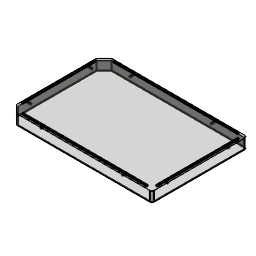
GREINER 96 WELL PLATE LID (Created) (Autodesk Fusion 360 design; units mm, degrees)
part number: 2026-02-05-10-27-23-618
Autodesk Fusion 360 part; units mm, degrees
sketch "Sketch1" plane through (0, 0, 0) normal (0, 0, 1) x (1, 0, 0)
  line L0 (61.42, -42.3) -> (-56.55, -42.3)
  line L1 (-63.55, -35.3) -> (-63.55, 35.3)
  line L2 (-56.55, 42.3) -> (61.42, 42.3)
  line L3 (63.55, 40.17) -> (63.55, -40.17)
  line L4 (63.55, -42.3) -> (-63.55, 42.3) construction
  line L5 (-63.55, -42.3) -> (63.55, 42.3) construction
  line L6 (-56.55, 42.3) -> (-63.55, 35.3)
  line L7 (0, -42.3) -> (0, 42.3) construction
  line L8 (63.55, 0) -> (-63.55, 0) construction
  line L9 (-56.55, -42.3) -> (-63.55, -35.3)
  arc A0 (63.55, 40.17) -> (61.42, 42.3) centre (61.42, 40.17) ccw
  arc A1 (61.42, -42.3) -> (63.55, -40.17) centre (61.42, -40.17) ccw
  dimension "d1" = 84.6
  dimension "d2" = 127.1
  dimension "d3" = 7
  dimension "d4" = 7
  dimension "d5" = 2.13
  constraint horizontal L0
  constraint perpendicular L0 L1
  constraint parallel L0 L2
  constraint parallel L1 L3
  constraint coincident L4 origin
  constraint coincident L5 origin
  constraint coincident L4.end L2
  constraint coincident L4.end L1
  constraint coincident L2 L7.end
  constraint perpendicular L2 L7
  constraint coincident L1 L8.end
  constraint perpendicular L1 L8
  constraint symmetric L2.start L8 L0.end
  constraint symmetric L1.end L8 L1.start
  constraint coincident L0 L7.start
  constraint coincident L3 L8.start
  constraint coincident L5.end L2
  constraint coincident L5.end L3
  constraint tangent L2 A0
  constraint tangent L3 A0
  constraint symmetric L8 L2.end L0.start
  constraint symmetric L8 L3.start L3.end
  constraint symmetric L8 A0 A1
  measures "d1" distance of L5.start L4.end
  measures "d2" distance of L4.end L5.end
  measures "d3" distance of L4.end L2.start
  measures "d4" distance of L4.end L1.end
  measures "d5" radius of A0
extrude "Extrude1" add sketch "Sketch1" against normal blind 9
sketch "Sketch2" plane through (0, 0, -9) normal (0, 0, -1) x (1, 0, 0)
  line L0 (61.42, 42.3) -> (-56.55, 42.3)
  line L1 (-56.55, 42.3) -> (-63.55, 35.3)
  line L2 (-63.55, 35.3) -> (-63.55, -35.3)
  line L3 (-63.55, -35.3) -> (-56.55, -42.3)
  line L4 (-56.55, -42.3) -> (61.42, -42.3)
  arc A0 (61.42, -42.3) -> (63.55, -40.17) centre (61.42, -40.17) ccw
  line L5 (63.55, -40.17) -> (63.55, 40.17)
  arc A1 (63.55, 40.17) -> (61.42, 42.3) centre (61.42, 40.17) ccw
  line L6 (61.42, -41.3) -> (-56.1358, -41.3)
  line L7 (-62.55, -34.8858) -> (-62.55, 34.8858)
  line L8 (-56.1358, 41.3) -> (61.42, 41.3)
  line L9 (62.55, 40.17) -> (62.55, -40.17)
  line L10 (62.55, -41.3) -> (-62.55, 41.3) construction
  line L11 (-62.55, -41.3) -> (62.55, 41.3) construction
  line L12 (-56.1358, 41.3) -> (-62.55, 34.8858)
  arc A2 (62.55, 40.17) -> (61.42, 41.3) centre (61.42, 40.17) ccw
  line L13 (63.55, 0) -> (-63.55, 0) construction
  line L14 (-56.1358, -41.3) -> (-62.55, -34.8858)
  arc A3 (61.42, -41.3) -> (62.55, -40.17) centre (61.42, -40.17) ccw
  dimension "d8" = 125.1
  dimension "d9" = 82.6
  dimension "d10" = 6.4142
  dimension "d11" = 6.4142
  dimension "d12" = 1
  dimension "d13" = 1.13
  constraint horizontal L6
  constraint perpendicular L6 L7
  constraint parallel L6 L8
  constraint parallel L7 L9
  constraint coincident L10 origin
  constraint coincident L11 origin
  constraint coincident L10.end L8
  constraint coincident L10.end L7
  constraint coincident L11.end L9
  constraint coincident L11.end L8
  constraint tangent L9 A2
  constraint tangent L8 A2
  constraint midpoint L5 L13.start
  constraint midpoint L2 L13.end
  constraint symmetric L8.start L13 L6.end
  constraint symmetric L7.end L13 L7.start
  constraint symmetric L9.start L13 L9.end
  constraint symmetric L8.end L13 L6.start
  constraint symmetric A2 L13 A3
  measures "d8" distance of L10.end L11.end
  measures "d9" distance of L11.start L10.end
  measures "d10" distance of L10.end L8.start
  measures "d11" distance of L10.end L7.end
  measures "d12" distance of L1 L12
  measures "d13" radius of A2
extrude "Extrude2" cut sketch "Sketch2" against normal blind 8 contours L6 L7 L8 L9 L12 A2 L14 A3
sketch "Sketch3" plane through (0, 0, -1) normal (0, 0, -1) x (1, 0, 0)
  line L0 (-56.1358, -41.3) -> (61.42, -41.3)
  arc A0 (61.42, -41.3) -> (62.55, -40.17) centre (61.42, -40.17) ccw
  line L1 (62.55, -40.17) -> (62.55, 40.17)
  arc A1 (62.55, 40.17) -> (61.42, 41.3) centre (61.42, 40.17) ccw
  line L2 (61.42, 41.3) -> (-56.1358, 41.3)
  line L3 (-56.1358, 41.3) -> (-62.55, 34.8858)
  line L4 (-62.55, 34.8858) -> (-62.55, -34.8858)
  line L5 (-62.55, -34.8858) -> (-56.1358, -41.3)
  line L6 (-62.55, 32.8642) -> (-35.55, 32.8642) construction
  line L7 (-35.55, 32.8642) -> (-35.55, 41.3) construction
  line L8 (-35.55, 41.3) -> (-36.55, 41.3)
  line L9 (-36.55, 41.3) -> (-36.55, 37.5)
  line L10 (-36.55, 37.5) -> (-35.55, 37.5)
  line L11 (-35.55, 37.5) -> (-35.55, 41.3)
  line L12 (-50.2731, 41.3) -> (-50.2731, 26.6) construction
  line L13 (-50.2731, 26.6) -> (-62.55, 26.6) construction
  line L14 (-62.55, 26.6) -> (-58.75, 26.6)
  line L15 (-58.75, 26.6) -> (-58.75, 27.6)
  line L16 (-58.75, 27.6) -> (-62.55, 27.6)
  line L17 (-62.55, 27.6) -> (-62.55, 26.6)
  line L18 (62.55, 0) -> (-62.55, 0) construction
  line L19 (-62.55, 30.673) -> (-62.55, 55) construction
  line L20 (62.55, 34.8173) -> (62.55, 55) construction
  line L21 (62.55, 55) -> (-62.55, 55) construction
  line L22 (0, 55) -> (0, -41.3) construction
  line L23 (62.55, 27.6) -> (62.55, 26.6)
  line L24 (62.55, 26.6) -> (58.75, 26.6)
  line L25 (58.75, 27.6) -> (62.55, 27.6)
  line L26 (58.75, 26.6) -> (58.75, 27.6)
  line L27 (36.55, 41.3) -> (36.55, 37.5)
  line L28 (35.55, 37.5) -> (35.55, 41.3)
  line L29 (36.55, 37.5) -> (35.55, 37.5)
  line L30 (35.55, 41.3) -> (36.55, 41.3)
  line L31 (62.55, -26.6) -> (58.75, -26.6)
  line L32 (58.75, -27.6) -> (62.55, -27.6)
  line L33 (58.75, -26.6) -> (58.75, -27.6)
  line L34 (35.55, -37.5) -> (35.55, -41.3)
  line L35 (36.55, -37.5) -> (35.55, -37.5)
  line L36 (36.55, -41.3) -> (36.55, -37.5)
  line L37 (62.55, -27.6) -> (62.55, -26.6)
  line L38 (35.55, -41.3) -> (36.55, -41.3)
  line L39 (-58.75, -26.6) -> (-58.75, -27.6)
  line L40 (-62.55, -26.6) -> (-58.75, -26.6)
  line L41 (-58.75, -27.6) -> (-62.55, -27.6)
  line L42 (-62.55, -27.6) -> (-62.55, -26.6)
  line L43 (-36.55, -37.5) -> (-35.55, -37.5)
  line L44 (-35.55, -37.5) -> (-35.55, -41.3)
  line L45 (-36.55, -41.3) -> (-36.55, -37.5)
  line L46 (-35.55, -41.3) -> (-36.55, -41.3)
  dimension "d16" = 27
  dimension "d17" = 3.8
  dimension "d18" = 1
  dimension "d19" = 14.7
  dimension "d20" = 3.8
  dimension "d21" = 1
  constraint coincident L4 L6.start
  constraint perpendicular L4 L6
  constraint coincident L2 L7.end
  constraint perpendicular L2 L7
  constraint horizontal L8
  constraint vertical L9
  constraint horizontal L10
  constraint vertical L11
  constraint coincident L2 L12.start
  constraint perpendicular L2 L12
  constraint coincident L4 L13.end
  constraint perpendicular L4 L13
  constraint horizontal L14
  constraint vertical L15
  constraint horizontal L16
  constraint vertical L17
  constraint midpoint L1 L18.start
  constraint midpoint L4 L18.end
  constraint coincident L4 L19.start
  constraint perpendicular L6 L19
  constraint coincident L1 L20.start
  constraint parallel L1 L20
  constraint perpendicular L19 L21
  constraint midpoint L21 L22.start
  constraint coincident L0 L22.end
  constraint perpendicular L0 L22
  constraint symmetric L7.end L22 L28.end
  constraint symmetric L8.end L22 L27.start
  constraint symmetric L9.end L22 L27.end
  constraint symmetric L10.end L22 L28.start
  constraint symmetric L13.end L22 L23.end
  constraint symmetric L14.end L22 L24.end
  constraint symmetric L15.end L22 L25.start
  constraint symmetric L16.end L22 L23.start
  constraint symmetric L7.end L18 L44.end
  constraint symmetric L8.end L18 L45.start
  constraint symmetric L9.end L18 L43.start
  constraint symmetric L10.end L18 L43.end
  constraint symmetric L13.end L18 L40.start
  constraint symmetric L14.end L18 L39.start
  constraint symmetric L15.end L18 L39.end
  constraint symmetric L16.end L18 L41.end
  constraint symmetric L18 L23.start L32.end
  constraint symmetric L18 L23.end L31.start
  constraint symmetric L18 L27.end L35.start
  constraint symmetric L18 L28.start L34.start
  constraint symmetric L18 L24.end L31.end
  constraint symmetric L18 L25.start L32.start
  constraint symmetric L18 L27.start L36.start
  constraint symmetric L18 L28.end L34.end
  measures "d16" distance of L6.start L6.end
  measures "d17" distance of L8.end L9.end
  measures "d18" distance of L9.end L10.end
  measures "d19" distance of L12.start L12.end
  measures "d20" distance of L15.end L16.end
  measures "d21" distance of L14.end L15.end
extrude "Extrude3" add sketch "Sketch3" along normal blind 1 contours L0 L43 L44 L45 L46 | L4 L39 L40 L41 L42 | L0 L34 L35 L36 L38 | L4 L14 L15 L16 L17 | L1 L31 L32 L33 L37 | L2 L8 L9 L10 L11 | L1 L23 L24 L25 L26 | L2 L27 L28 L29 L30
sketch "Sketch4" plane through (0, 0, 0) normal (0, 0, 1) x (-1, 0, 0)
  line L0 (56.55, 42.3) -> (-61.42, 42.3)
  arc A0 (-61.42, 42.3) -> (-63.55, 40.17) centre (-61.42, 40.17) ccw
  line L1 (-63.55, 40.17) -> (-63.55, -40.17)
  arc A1 (-63.55, -40.17) -> (-61.42, -42.3) centre (-61.42, -40.17) ccw
  line L2 (-61.42, -42.3) -> (56.55, -42.3)
  line L3 (56.55, -42.3) -> (63.55, -35.3)
  line L4 (63.55, -35.3) -> (63.55, 35.3)
  line L5 (63.55, 35.3) -> (56.55, 42.3)
  line L6 (-63.55, -34.3916) -> (-62.25, -34.3916) construction
  line L7 (-62.25, -34.3916) -> (-62.25, -36.4) construction
  line L8 (-60, -42.3) -> (-66.2, -42.3) construction
  line L9 (-63.55, -39.2433) -> (-63.55, -43.1) construction
  line L10 (-62.25, -36.4) -> (-60.95, -36.4)
  line L11 (-60.95, -36.4) -> (-60.95, 36.4)
  line L12 (-60.95, 36.4) -> (-62.25, 36.4)
  line L13 (-62.25, 36.4) -> (-62.25, -36.4)
  line L14 (-52.6219, -42.3) -> (-52.6219, -41) construction
  line L15 (-52.6219, -41) -> (-57.65, -41) construction
  line L16 (-57.65, -41) -> (53.05, -41)
  line L17 (53.05, -41) -> (53.05, -39.7)
  line L18 (53.05, -39.7) -> (-57.65, -39.7)
  line L19 (-57.65, -39.7) -> (-57.65, -41)
  line L20 (53.05, 39.7) -> (-57.65, 39.7)
  line L21 (-57.65, 41) -> (53.05, 41)
  line L22 (-57.65, 39.7) -> (-57.65, 41)
  line L23 (53.05, 41) -> (53.05, 39.7)
  line L24 (60.95, 0) -> (60.95, -32.3)
  line L25 (60.95, -32.3) -> (62.25, -32.3)
  line L26 (62.25, -32.3) -> (62.25, 0)
  line L27 (60.95, 0) -> (60.95, 32.3)
  line L28 (62.25, 32.3) -> (62.25, 0)
  line L29 (60.95, 32.3) -> (62.25, 32.3)
  line L30 (-63.55, 0) -> (60.95, 0) construction
  line L31 (62.25, 0) -> (63.55, 0) construction
  dimension "d24" = 1.3
  dimension "d25" = 5.9
  dimension "d26" = 72.8
  dimension "d27" = 1.3
  dimension "d28" = 1.3
  dimension "d29" = 5.9
  dimension "d30" = 1.3
  dimension "d31" = 110.7
  dimension "d32" = 32.3
  dimension "d33" = 1.3
  dimension "d34" = 1.3
  constraint coincident L1 L6.start
  constraint perpendicular L1 L6
  constraint perpendicular L6 L7
  constraint coincident L2 L8.start
  constraint parallel L2 L8
  constraint coincident L1 L9.start
  constraint perpendicular L2 L9
  constraint horizontal L10
  constraint vertical L11
  constraint horizontal L12
  constraint vertical L13
  constraint coincident L2 L14.start
  constraint perpendicular L2 L14
  constraint perpendicular L14 L15
  constraint horizontal L16
  constraint vertical L17
  constraint horizontal L18
  constraint vertical L19
  constraint midpoint L1 L30.start
  constraint midpoint L4 L31.end
  constraint symmetric L15.end L21.start L30
  constraint symmetric L16.end L21.end L30
  constraint symmetric L17.end L20.start L30
  constraint symmetric L18.end L20.end L30
  constraint vertical L24
  constraint horizontal L25
  constraint vertical L26
  constraint symmetric L24.end L27.end L30
  constraint symmetric L25.end L28.start L31
  constraint collinear L30 L31
  measures "d24" distance of L6.start L6.end
  measures "d25" distance of L7.end L8
  measures "d26" distance of L10.end L11.end
  measures "d27" distance of L7.end L10.end
  measures "d28" distance of L14.start L14.end
  measures "d29" distance of L9 L15.end
  measures "d30" distance of L15.end L18.end
  measures "d31" distance of L17.end L18.end
  measures "d32" distance of L24.start L24.end
  measures "d33" distance of L24.end L25.end
  measures "d34" distance of L4 L26
extrude "Extrude4" add sketch "Sketch4" along normal blind 1 contours L10 L11 L12 L13 | L16 L17 L18 L19 | L20 L21 L22 L23 | L24 L25 L26 L27 L28 L29
equation "d4 = d3"
equation "d11 = d10"
